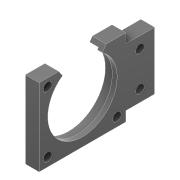
# Autodesk Inventor part: LargeLensHolderP1S2
Saved by Autodesk Inventor 2022 (Build 260153000, 153)
## iProperties
Created: 2021-12-05
Part Number: LargeLensHolderP1S2
Material: Acetal Resin, Black
Document SubType Name: Modeling
Designer: eganc
Density: 1.425 g/cm^3
Appearance: Smooth - Black
Author: eganc
Autodesk Inventor part; units mm, degrees
ref_plane "YZ Plane" through (0, 0, 0) normal (1, 0, 0) x (0, 1, 0)
ref_plane "XZ Plane" through (0, 0, 0) normal (0, 1, 0) x (-1, 0, 0)
sketch "Sketch1" plane through (0, 0, 0) normal (1, 0, 0) x (0, 1, 0)
  line L0 (-15, 15) -> (15, 15)
  line L1 (15, 15) -> (15, -15)
  line L2 (15, -15) -> (-15, -15)
  line L3 (-15, -15) -> (-15, 15)
  line L4 (-15, 15) -> (15, -15) construction
  line L5 (15, 15) -> (-15, -15) construction
  point P0 (0, 0)
  dimension "d0" = 30
  dimension "d1" = 30
  constraints: 12 end point, 2 midpoint, 2 parallel, 1 horizontal, 1 perpendicular
  measures "d0" distance of L0.end L1.end
  measures "d1" distance of L1.end L2.end
extrude "Extrusion1" add sketch "Sketch1" along normal blind 1.7695
sketch "Sketch2" plane through (1.7695, 0, 0) normal (1, 0, 0) x (0, 0, -1)
  circle A0 centre (0, 0) radius 12
  dimension "d4" = 24
  constraints: 1 centre point, 1 coincident
  measures "d4" diameter of A0
extrude "Extrusion2" cut sketch "Sketch2" against normal up to next
sketch "Sketch3" plane through (0, 0, 0) normal (0, 0, 1) x (1, 0, 0)
  line L0 (1.7695, 15) -> (1.7695, -15) projected
  line L1 (1.7695, 0) -> (1.7695, -12.5584)
  line L2 (0.5, 0) -> (1.7695, 0)
  arc A0 (0.5, 0) -> (1.7695, -12.5584) centre (63.25, 0) ccw
  point P0 (0, 0)
  dimension "d7" = 12.5584
  dimension "d8" = 125.5
  constraints: 4 end point, 2 point on circle, 2 point on line, 1 centre point, 1 horizontal, 1 midpoint
  measures "d7" distance of L1.start L1.end
  measures "d8" diameter of A0
revolve "Revolution1" cut sketch "Sketch3" angle 360 about axis through (0.5, 0, 0) along (1, 0, 0)
sketch "Sketch4" plane through (1.7695, 0, 0) normal (1, 0, 0) x (0, 0, -1)
  circle A0 centre (0, 0) radius 12.7
  line L0 (-15, 15) -> (-15, -15) projected
  line L1 (-15, 15) -> (15, 15)
  line L2 (15, 15) -> (15, -15)
  line L3 (15, -15) -> (-15, -15)
  line L4 (-15, -15) -> (-15, 15)
  dimension "d10" = 25.4
  constraints: 8 end point, 2 coincident, 2 parallel, 1 centre point, 1 horizontal, 1 perpendicular
  measures "d10" diameter of A0
extrude "Extrusion3" add sketch "Sketch4" along normal blind 3
ref_plane "Work Plane1" through (0, 0, 0) normal (-1, 0, 0) x (0, 0, 1)
mirror "Mirror1" about plane through (0, 0, 0) normal (-1, 0, 0) of "Extrusion1", "Extrusion2", "Revolution1", "Extrusion3"
sketch "Sketch8" plane through (4.7695, 0, 0) normal (1, 0, 0) x (0, 0, -1)
  circle A0 centre (12, -12) radius 1.5
  line L0 (-15, -15) -> (15, -15) projected
  line L1 (15, -15) -> (15, 15) projected
  circle A1 centre (-12, -12) radius 1.5
  circle A2 centre (-12, 9) radius 1.5
  line L2 (-15, 15) -> (-15, -15) projected
  line L3 (15, 15) -> (-15, 15) projected
  point P0 (0, 0)
  dimension "d30" = 3
  dimension "d31" = 3
  dimension "d32" = 3
  dimension "d33" = 3
  dimension "d34" = 3
  dimension "d35" = 3
  dimension "d36" = 6
  constraints: 3 centre point, 2 equal radius
  measures "d30" diameter of A0
  measures "d31" distance from line of L0 A0.centre
  measures "d32" distance from line of L1 A0.centre
  measures "d33" distance from line of L0 A1.centre
  measures "d34" distance from line of L2 A1.centre
  measures "d35" distance from line of L2 A2.centre
  measures "d36" distance from line of L3 A2.centre
extrude "Extrusion7" cut sketch "Sketch8" against normal up to surface (9.5391 mm away) contours A0 | A1 | A2
sketch "Sketch9" plane through (4.7695, 0, 0) normal (1, 0, 0) x (0, 0, -1)
  line L0 (0, 0) -> (-8.2274, 11.75)
  line L1 (-8.2274, 11.75) -> (-15, 11.75)
  line L2 (-15, 15) -> (-15, -15) projected
  line L3 (0, 0) -> (0, 15) construction
  line L4 (-15, 11.75) -> (-15, 15)
  line L5 (15, 15) -> (-15, 15) projected
  line L6 (0, 15) -> (-15, 15)
  line L7 (0, 0) -> (8.2274, 11.75)
  line L8 (8.2274, 11.75) -> (15, 11.75)
  line L9 (15, 15) -> (15, -15)
  line L10 (-15, 15) -> (15, 15)
  dimension "d39" = 35
  dimension "d42" = 3.25
  constraints: 18 end point, 5 symmetric about line, 2 horizontal, 2 point on line, 1 collinear, 1 vertical
  measures "d39" angle of L3 L0
  measures "d42" distance between parallel lines of L5 L1
extrude "Extrusion8" cut sketch "Sketch9" against normal up to surface (9.5391 mm away)
sketch "Sketch11" plane through (4.7695, -15, -15) normal (0, 0, -1) x (-1, 0, 0)
  line L0 (9.5391, 0) -> (9.5391, 26.75) projected
  line L1 (0, 0) -> (9.5391, 26.75) construction
  line L2 (0, 26.75) -> (9.5391, 26.75) projected
  line L3 (0, 26.75) -> (9.5391, 0) construction
  line L4 (0, 0) -> (0, 26.75) projected
  line L5 (9.5391, 3.375) -> (0, 3.375)
  line L6 (0, 3.375) -> (0, 23.375)
  line L7 (0, 23.375) -> (9.5391, 23.375)
  line L8 (9.5391, 23.375) -> (9.5391, 3.375)
  line L9 (9.5391, 3.375) -> (0, 23.375) construction
  line L10 (0, 3.375) -> (9.5391, 23.375) construction
  point P0 (4.7695, 15)
  point P1 (4.7695, 13.375)
  dimension "d46" = 20
  constraints: 16 end point, 3 midpoint, 2 parallel, 1 horizontal, 1 perpendicular, 1 point on line
  measures "d46" distance between parallel lines of L7 L5
extrude "Extrusion10" add sketch "Sketch11" along normal blind 10 contours L5 L4 L7 L0
sketch "Sketch12" plane through (-4.7695, -15, -15) normal (-1, 0, 0) x (0, 0, 1)
  circle A0 centre (-5, 19.375) radius 1.5
  circle A1 centre (-5, 7.375) radius 1.5
  line L0 (0, 3.375) -> (-10, 3.375) projected
  line L1 (0, 23.375) -> (-10, 23.375) projected
  point P0 (15, 15)
  dimension "d49" = 4
  dimension "d50" = 5
  dimension "d51" = 4
  dimension "d52" = 5
  dimension "d53" = 3
  constraints: 2 centre point, 1 equal radius
  measures "d49" distance from line of L0 A1.centre
  measures "d50" horizontal distance of L0.start A1.centre
  measures "d51" distance from line of L1 A0.centre
  measures "d52" horizontal distance of L1.start A0.centre
  measures "d53" diameter of A0
extrude "Extrusion11" cut sketch "Sketch12" against normal up to surface (9.5391 mm away)
sketch "Sketch13" plane through (4.7695, -15, -15) normal (0, -1, 0) x (1, 0, 0)
  line L0 (-9.5391, 30) -> (0, 30) projected
  line L1 (-4.7695, 30) -> (-4.7695, -10)
  line L2 (0, -10) -> (-9.5391, -10) projected
  point P0 (-4.7695, 15)
  constraints: 2 end point, 2 midpoint
split body "Split2" sketch "Sketch13" result one side removed curves L1 removed pieces at (0.5, -13.971, -0.4809)
equation "\"d37\" = d32"
body "Solid1"
